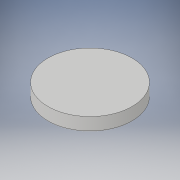
# Autodesk Inventor part: stem
Saved by Autodesk Inventor 2019 (Build 230136000, 136)
## iProperties
Created: 2019-02-27
Part Number: stem
Material: Generic
Document SubType Name: Modeling
Designer: jmc
Density: 1 g/cm^3
Appearance: Default
Author: jmc
Autodesk Inventor part; units mm, degrees
ref_plane "YZ Plane" through (0, 0, 0) normal (1, 0, 0) x (0, 1, 0)
ref_plane "XZ Plane" through (0, 0, 0) normal (0, 1, 0) x (-1, 0, 0)
ref_plane "XY Plane" through (0, 0, 0) normal (0, 0, 1) x (1, 0, 0)
sketch "Sketch1" plane through (0, 0, 0) normal (0, 1, 0) x (-1, 0, 0)
  circle A0 centre (0, 0) radius 9.08
  dimension "d0" = 18.16
  constraints: 1 centre point, 1 coincident
  measures "d0" diameter of A0
extrude "Extrusion1" add sketch "Sketch1" along normal blind 1
sketch "Sketch2" plane through (0, 0, 0) normal (0, -1, 0) x (1, 0, 0)
  circle A0 centre (0, 0) radius 7.265
  dimension "d3" = 14.53
  constraints: 1 centre point, 1 coincident
  measures "d3" diameter of A0
extrude "Extrusion2" [suppressed]
sketch "Sketch5" plane through (0, 0, 0) normal (0, 0, 1) x (1, 0, 0)
  line L0 (9.08, 0) -> (9.08, 1) projected
  line L1 (9.08, 0) -> (9.08, -1.6895)
  line L2 (-9.08, 0) -> (9.08, 0) projected
  line L3 (-9.08, 0) -> (-9.08, -1.6895)
  arc A0 (8.7986, -1.8721) -> (-8.7986, -1.8721) centre (0, -21.6116) ccw
  arc A1 (-9.08, -1.6895) -> (-8.7986, -1.8721) centre (-8.88, -1.6895) ccw
  arc A2 (8.7986, -1.8721) -> (9.08, -1.6895) centre (8.88, -1.6895) ccw
  line L4 (0, -26.3403) -> (0, 6.7607) projected
  point P0 (0, 0)
  point P1 (9.08, -2)
  point P2 (-9.08, -2)
  dimension "d7" = 2
  dimension "d8" = 2
  dimension "d9" = 0.2
  dimension "d10" = 0.2
  constraints: 9 point on circle, 4 end point, 4 tangent, 3 centre point, 3 point on line, 1 collinear, 1 vertical
  measures "d7" distance of L1.start point (9.08, -2)
  measures "d8" distance of L2.start point (-9.08, -2)
  measures "d9" radius of A1
  measures "d10" radius of A2
revolve "Revolution1" add sketch "Sketch5" angle 360 about axis through (0, -10, 0) along (0, 1, 0) contours L1 A2 A0 L2
body "Solid1"
